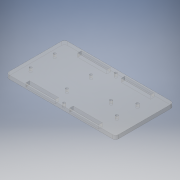
# Autodesk Inventor part: Interrupter_Bottom
Saved by Autodesk Inventor 2016 (Build 200138000, 138)
## iProperties
Created: 2018-05-24
Part Number: Interrupter_Bottom
Material: Polycarbonate, Clear
Document SubType Name: Modeling
Designer: Phil Erle
Density: 1.2 g/cm^3
Appearance: Polycarbonate - Clear
Author: Phil Erle
Autodesk Inventor part; units mm, degrees
ref_plane "YZ Plane" through (0, 0, 0) normal (1, 0, 0) x (0, 1, 0)
ref_plane "XZ Plane" through (0, 0, 0) normal (0, 1, 0) x (-1, 0, 0)
ref_plane "XY Plane" through (0, 0, 0) normal (0, 0, 1) x (1, 0, 0)
sketch "Sketch1" plane through (0, 0, 0) normal (0, 0, 1) x (1, 0, 0)
  line L0 (-75, -40) -> (75, -40)
  line L1 (75, -40) -> (75, 40)
  line L2 (75, 40) -> (-75, 40)
  line L3 (-75, 40) -> (-75, -40)
  line L4 (-75, -40) -> (75, 40) construction
  line L5 (75, -40) -> (-75, 40) construction
  point P0 (0, 0)
  dimension "d0" = 80
  dimension "d1" = 150
  constraints: 12 end point, 2 midpoint, 2 parallel, 1 horizontal, 1 perpendicular
  measures "d0" distance of L0.end L1.end
  measures "d1" distance of L1.end L2.end
extrude "Extrusion1" add sketch "Sketch1" along normal blind 5
sketch "Sketch2" plane through (0, 0, 5) normal (0, 0, 1) x (1, 0, 0)
  line L0 (29, -14.15) -> (51, -14.15) construction
  line L1 (51, -14.15) -> (51, 14.15) construction
  line L2 (51, 14.15) -> (29, 14.15) construction
  line L3 (29, 14.15) -> (29, -14.15) construction
  line L4 (29, -14.15) -> (51, 14.15) construction
  line L5 (51, -14.15) -> (29, 14.15) construction
  line L6 (-65, -16.5) -> (-15, -16.5) construction
  line L7 (-15, -16.5) -> (-15, 16.5) construction
  line L8 (-15, 16.5) -> (-65, 16.5) construction
  line L9 (-65, 16.5) -> (-65, -16.5) construction
  line L10 (-65, -16.5) -> (-15, 16.5) construction
  line L11 (-15, -16.5) -> (-65, 16.5) construction
  point P0 (0, 0)
  point P1 (40, 0)
  point P2 (-40, 0)
  point P3 (-40, 0)
  point P4 (40, 0)
  point P5 (29, 0)
  dimension "d4" = 50
  dimension "d5" = 33
  dimension "d6" = 40
  dimension "d7" = 28.3
  dimension "d8" = 22
  dimension "d9" = 40
  constraints: 24 end point, 7 midpoint, 6 coincident, 4 parallel, 2 horizontal, 2 horizontal alignment, 2 perpendicular
  measures "d4" distance of L8.end L7.end
  measures "d5" distance of L7.end L6.end
  measures "d6" distance of point (0, 0) point (-40, 0)
  measures "d7" distance of L0.end L1.end
  measures "d8" distance of L1.end L2.end
  measures "d9" distance of point (0, 0) point (40, 0)
hole "Hole1" at (51, 14.15, 5) at (51, -14.15, 5) at (29, 0, 5) at (-15, -16.5, 5) at (-15, 16.5, 5) at (-65, 16.5, 5) at (-65, -16.5, 5) direction (0, 0, -1) diameter 3.4 depth 8 tip angle 118 clearance for "Countersunk Flat Head Screw DIN EN ISO 2009" size "M3" standard "DIN"
sketch "Sketch3" plane through (0, 0, 5) normal (0, 0, 1) x (1, 0, 0)
  line L0 (-50, 38) -> (50, 38) construction
  line L1 (50, 38) -> (50, 33) construction
  line L2 (50, 33) -> (-50, 33) construction
  line L3 (-50, 33) -> (-50, 38) construction
  line L4 (-50, 38) -> (50, 33) construction
  line L5 (50, 38) -> (-50, 33) construction
  line L6 (-50, -33) -> (50, -33) construction
  line L7 (50, -33) -> (50, -38) construction
  line L8 (50, -38) -> (-50, -38) construction
  line L9 (-50, -38) -> (-50, -33) construction
  line L10 (-50, -33) -> (50, -38) construction
  line L11 (50, -33) -> (-50, -38) construction
  line L12 (75, 40) -> (-75, 40) projected
  line L13 (-75, -40) -> (75, -40) projected
  line L14 (-50, 38) -> (-10, 38)
  line L15 (-10, 38) -> (-10, 33)
  line L16 (-10, 33) -> (-50, 33)
  line L17 (-50, 33) -> (-50, 38)
  line L18 (50, 38) -> (10, 38)
  line L19 (10, 38) -> (10, 33)
  line L20 (10, 33) -> (50, 33)
  line L21 (50, 33) -> (50, 38)
  line L22 (50, -33) -> (10, -33)
  line L23 (10, -33) -> (10, -38)
  line L24 (10, -38) -> (50, -38)
  line L25 (50, -38) -> (50, -33)
  line L26 (-50, -33) -> (-10, -33)
  line L27 (-10, -33) -> (-10, -38)
  line L28 (-10, -38) -> (-50, -38)
  line L29 (-50, -38) -> (-50, -33)
  point P0 (0, 0)
  point P1 (0, 35.5)
  point P2 (0, -35.5)
  point P3 (0, 35.5)
  point P4 (0, -35.5)
  dimension "d17" = 5
  dimension "d18" = 5
  dimension "d19" = 2
  dimension "d20" = 2
  dimension "d21" = 100
  dimension "d22" = 20
  dimension "d23" = 10
  constraints: 56 end point, 12 parallel, 6 horizontal, 6 midpoint, 6 perpendicular, 5 point on line, 4 vertical alignment
  measures "d17" distance of L2.end L0.start
  measures "d18" distance of L8.end L6.start
  measures "d19" distance between parallel lines of L12 L0
  measures "d20" distance between parallel lines of L13 L8
  measures "d21" distance of L0.start L0.end
  measures "d22" distance between parallel lines of L19 L15
  measures "d23" distance from line of point (0, 0) L15
extrude "Extrusion2" cut sketch "Sketch3" against normal blind 5
fillet "Fillet1" radius 4 4 edges at (75, 40, 2.5) (75, -40, 2.5) (-75, -40, 2.5) (-75, 40, 2.5)
sketch "Sketch4" plane through (0, 0, 5) normal (0, 0, 1) x (1, 0, 0)
  line L0 (-10, -38) -> (-50, -38) projected
  line L1 (-50, 38) -> (-10, 38) projected
  point P0 (0, 0)
  point P1 (0, 35.5)
  point P2 (0, -35.5)
  dimension "d27" = 2.5
  dimension "d28" = 2.5
  constraints: 2 vertical alignment
  measures "d27" distance from line of point (0, -35.5) L0
  measures "d28" distance from line of point (0, 35.5) L1
hole "Hole2" at (0, 35.5, 5) at (0, -35.5, 5) direction (0, 0, -1) diameter 3.4 depth 8 tip angle 118 clearance for "Countersunk Flat Head Screw DIN EN ISO 2009" size "M3" standard "DIN"
equation "\"d23\" = 0.5 * d22"
body "Solid1"
